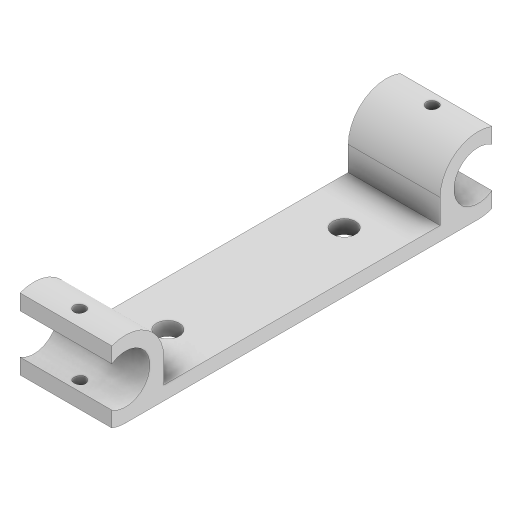
# Autodesk Inventor part: pipe_holder_typeB
Saved by Autodesk Inventor 2023 (Build 270158000, 158)
## iProperties
Created: 2024-07-05
Part Number: pipe_holder_typeB
Material: 일반
Document SubType Name: Modeling
Designer: Gihyeok Na
Density: 1 g/cm^3
Appearance: 기본값
Author: Gihyeok Na
Autodesk Inventor part; units mm, degrees
ref_plane "YZ Plane" through (0, 0, 0) normal (1, 0, 0) x (0, 1, 0)
ref_plane "XZ Plane" through (0, 0, 0) normal (0, 1, 0) x (-1, 0, 0)
sketch "스케치1" plane through (0, 0, 0) normal (1, 0, 0) x (0, 1, 0)
  circle A0 centre (0, 0) radius 5.3
  circle A1 centre (0, 0) radius 5
  line L0 (4, 3) -> (-4, 3)
  circle A2 centre (0, 0) radius 8.3
  line L1 (4, 3) -> (11.6093, 3)
  line L2 (-4, 3) -> (-10.334, 3)
  line L3 (11.6093, -38.4) -> (-10.334, -38.4) construction
  circle A3 centre (0, -76.8) radius 5.3
  circle A4 centre (0, -76.8) radius 5
  line L4 (4, -79.8) -> (-4, -79.8)
  circle A5 centre (0, -76.8) radius 8.3
  line L5 (4, -79.8) -> (11.6093, -79.8)
  line L6 (-4, -79.8) -> (-10.334, -79.8)
  line L7 (-8.3, 0) -> (-8.3, -76.8)
  line L8 (-5.3, 0) -> (-5.3, -76.8)
  line L9 (0, -8.3) -> (-5.3, -8.3)
  line L10 (0, -68.5) -> (-5.3, -68.5)
  point P0 (0, 3)
  point P1 (0, -79.8)
  point P2 (-4.3692, -79.8)
  point P3 (4.3692, -79.8)
  point P4 (7.7389, 3)
  point P5 (4.3692, 3)
  point P6 (-4.3692, 3)
  point P7 (-7.7389, 3)
  point P8 (-7.7389, -79.8)
  point P9 (7.7389, -79.8)
  dimension "d0" = 10.6
  dimension "d1" = 3
  dimension "d2" = 10
  dimension "d3" = 16.6
  dimension "d4" = 38.4
  constraints: 22 end point, 11 symmetric about line, 6 coincident, 6 point on circle, 5 horizontal, 3 centre point, 2 vertical, 1 perpendicular, 1 point on line, 11 other
  measures "d1" distance of point (0, 3) point (0, 0)
  measures "d2" diameter of A1
  measures "d3" diameter of A2
  measures "d4" distance from line of L3 point (0, 0)
extrude "돌출1" add sketch "스케치1" along normal blind 20 contours L8 A2 L2 A0 | A0 L1 A2 L8 | L8 A5 L7 A2 | A2 L9 L8 | A5 L8 A3 L6 | L10 A5 L8 | A5 L5 A3 L8
ref_plane "작업 평면1" through (0, 0, 8.3) normal (0, 0, 1) x (1, 0, 0)
sketch "스케치3" plane through (0, -8.3, -76.8) normal (0, -1, 0) x (1, 0, 0)
  line L0 (0, 76.8) -> (0, 0) projected
  line L1 (0, 0) -> (20, 0) projected
  line L2 (20, 76.8) -> (20, 0) projected
  line L3 (0, 76.8) -> (20, 76.8) projected
  line L4 (0, 0) -> (0, -3) projected
  line L5 (0, -3) -> (20, -3) projected
  line L6 (20, 0) -> (20, -3) projected
  line L7 (0, 0) -> (20, 0) projected
  line L8 (0, 79.8) -> (0, 76.8) projected
  line L9 (0, 76.8) -> (20, 76.8) projected
  line L10 (20, 79.8) -> (20, 76.8) projected
  line L11 (0, 79.8) -> (20, 79.8) projected
  line L12 (20, 38.4) -> (0, 38.4) construction
  line L13 (0, 79.8) -> (20, 79.8) projected
  line L14 (10, 79.8) -> (10, -3) construction
  circle A0 centre (10, 19.2) radius 2.5
  line L15 (6, 12.3) -> (14, 12.3)
  line L16 (14, 12.3) -> (14, 4.3)
  line L17 (14, 4.3) -> (6, 4.3)
  line L18 (6, 4.3) -> (6, 12.3)
  line L19 (0, 8.3) -> (20, 8.3) projected
  line L20 (6, 12.3) -> (14, 4.3) construction
  line L21 (14, 12.3) -> (6, 4.3) construction
  circle A1 centre (10, 57.6) radius 2.5
  line L22 (6, 64.5) -> (14, 64.5)
  line L23 (14, 64.5) -> (14, 72.5)
  line L24 (14, 72.5) -> (6, 72.5)
  line L25 (6, 72.5) -> (6, 64.5)
  line L26 (0, 68.5) -> (20, 68.5)
  line L27 (6, 64.5) -> (14, 72.5) construction
  line L28 (14, 64.5) -> (6, 72.5) construction
  circle A2 centre (10, 0) radius 1.25
  circle A3 centre (10, 76.8) radius 1.25
  point P0 (10, 8.3)
  point P1 (10, 68.5)
  dimension "d10" = 38.4
  dimension "d11" = 10
  dimension "d12" = 5
  dimension "d13" = 19.2
  dimension "d14" = 8
  dimension "d15" = 8
  dimension "d20" = 2.5
  constraints: 30 end point, 9 symmetric about line, 8 midpoint, 4 centre point, 2 horizontal, 2 parallel, 2 point on line, 1 perpendicular, 1 vertical, 2 other
  measures "d10" distance between parallel lines of L1 L12
  measures "d11" distance between parallel lines of L14 L2
  measures "d12" diameter of A0
  measures "d13" distance from line of A0.centre L12
  measures "d14" distance of L16.end L17.end
  measures "d15" distance of L15.end L16.end
  measures "d20" diameter of A2
extrude "돌출3" cut sketch "스케치3" against normal blind 20 contours A3 L3 | L3 A3 | A2 L1 | L1 A2 | A0 | A1
extrude "돌출4" add sketch "스케치3" along normal blind 2 contours L26 L23 L22 L25 | L25 L24 L23 L26 | L19 L16 L17 L18 | L18 L15 L16 L19
